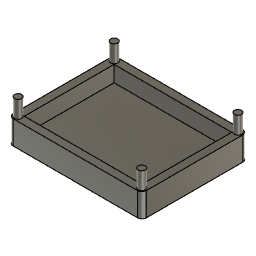
_part 2.99b838c8-83c5-4aec-84e9-91cd62201415 (Autodesk Fusion 360 design; units mm, degrees)
Autodesk Fusion 360 part; units mm, degrees
sketch "Sketch1" plane through (0, 0, 0) normal (0, 0, 1) x (1, 0, 0)
  line L0 (-15.5, 12.25) -> (15.5, 12.25)
  line L1 (15.5, 12.25) -> (15.5, -12.25)
  line L2 (15.5, -12.25) -> (-15.5, -12.25)
  line L3 (-15.5, -12.25) -> (-15.5, 12.25)
  line L4 (-15.5, 12.25) -> (15.5, -12.25) construction
  line L5 (15.5, 12.25) -> (-15.5, -12.25) construction
  dimension "d1" = 31
  dimension "d2" = 24.5
  constraint horizontal L0
  constraint perpendicular L0 L1
  constraint parallel L0 L2
  constraint parallel L1 L3
  constraint coincident L4 origin
  constraint coincident L5 origin
  measures "d1" distance of L0.start L0.end
  measures "d2" distance of L0.start L2.end
extrude "Extrude1" add sketch "Sketch1" along normal blind 5.5
shell "Shell1" thickness 1.8 removed faces 1 at (-5.1667, 4.0833, 5.5)
sketch "Sketch2" plane through (0, 0, 5.5) normal (0, 0, 1) x (-1, 0, 0)
  line L0 (13.7, 10.45) -> (13.7, -10.45)
  line L1 (13.7, -10.45) -> (-13.7, -10.45)
  line L2 (-13.7, -10.45) -> (-13.7, 10.45)
  line L3 (-13.7, 10.45) -> (13.7, 10.45)
  line L4 (15.5, 12.25) -> (-15.5, 12.25)
  line L5 (-15.5, 12.25) -> (-15.5, -12.25)
  line L6 (-15.5, -12.25) -> (15.5, -12.25)
  line L7 (15.5, -12.25) -> (15.5, 12.25)
  circle A0 centre (14.4, -11.2) radius 0.84
  line L8 (0, 0) -> (0, -2)
  line L9 (0, 0) -> (4, 0)
  circle A1 centre (-14.4, -11.2) radius 0.84
  circle A2 centre (-14.4, 11.2) radius 0.84
  circle A3 centre (14.4, 11.2) radius 0.84
  dimension "d6" = 1.68
  dimension "d7" = 11.2
  dimension "d8" = 14.4
  constraint coincident L8.start L9.start
  constraint vertical L8
  constraint perpendicular L8 L9
  constraint symmetric A0 L8 A1
  constraint symmetric A0 L9 A3
  constraint symmetric L9 A1 A2
  measures "d6" diameter of A0
  measures "d7" vertical distance of L8.start A0.centre
  measures "d8" horizontal distance of L8.start A0.centre
extrude "Extrude2" add sketch "Sketch2" along normal blind 4 contours A0 | A1 | A2 | A3
fillet "Fillet1" radius 1 1 edges at (15.5, -12.25, 2.75)
fillet "Fillet1" radius 1 1 edges at (15.5, 12.25, 2.75)
fillet "Fillet1" radius 1 1 edges at (-15.5, 12.25, 2.75)
fillet "Fillet1" radius 1 1 edges at (-15.5, -12.25, 2.75)
